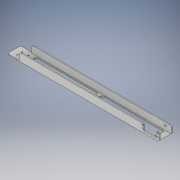
# Autodesk Inventor part: ArmProto1.2
Saved by Autodesk Inventor 2017 (Build 210142000, 142)
## iProperties
Created: 2017-09-30
Part Number: ArmProto1.2
Material: Generic
Document SubType Name: Modeling
Designer: User
Density: 1 g/cm^3
Appearance: Default
Author: User
Autodesk Inventor part; units mm, degrees
ref_plane "YZ Plane" through (0, 0, 0) normal (1, 0, 0) x (0, 1, 0)
ref_plane "XZ Plane" through (0, 0, 0) normal (0, 1, 0) x (-1, 0, 0)
ref_plane "XY Plane" through (0, 0, 0) normal (0, 0, 1) x (1, 0, 0)
sketch "Sketch1" plane through (0, 0, 0) normal (1, 0, 0) x (0, 1, 0)
  line L0 (0, 0) -> (25.4, 0)
  line L1 (25.4, 0) -> (25.4, -42.799)
  line L2 (25.4, -42.799) -> (0, -42.799)
  line L3 (0, -42.799) -> (0, 0)
  line L4 (25.4, -3.175) -> (3.175, -3.175)
  line L5 (3.175, -3.175) -> (3.175, -39.624)
  line L6 (3.175, -39.624) -> (25.4, -39.624)
  line L7 (25.4, -39.624) -> (25.4, -3.175)
  dimension "d0" = 25.4
  dimension "d1" = 42.799
  dimension "d2" = 22.225
  dimension "d3" = 36.449
  dimension "d4" = 3.175
  constraints: 16 end point, 4 parallel, 2 horizontal, 2 perpendicular, 1 point on line
  measures "d0" distance of L1.end L2.end
  measures "d1" distance of L0.end L1.end
  measures "d2" distance of L5.end L6.end
  measures "d3" distance of L4.end L5.end
  measures "d4" distance between parallel lines of L0 L4
extrude "Extrusion1" add sketch "Sketch1" along normal blind 495.3 contours L0 L1 L4 L5 L6 L2 L3
sketch "Sketch2" plane through (0, 0, 0) normal (0, 0, 1) x (1, 0, 0)
  line L0 (0, 25.4) -> (0, 0) projected
  line L1 (0, 0) -> (495.3, 0) projected
  line L2 (495.3, 25.4) -> (495.3, 0) projected
  line L3 (0, 25.4) -> (495.3, 25.4) projected
  line L4 (486.41, 25.4) -> (444.5, 25.4)
  line L5 (444.5, 25.4) -> (444.5, 6.35)
  line L6 (444.5, 6.35) -> (486.41, 6.35)
  line L7 (486.41, 6.35) -> (486.41, 25.4)
  circle A0 centre (490.2962, 21.2344) radius 2.413
  circle A1 centre (490.2962, 11.2344) radius 2.413
  circle A2 centre (440.7962, 21.2344) radius 2.413
  circle A3 centre (440.7962, 11.2344) radius 2.413
  dimension "d7" = 8.89
  dimension "d8" = 25.4
  dimension "d9" = 19.05
  dimension "d10" = 50.8
  dimension "d11" = 4.826
  dimension "d12" = 4.826
  dimension "d13" = 4.1656
  dimension "d14" = 10
  dimension "d15" = 4.826
  dimension "d16" = 4.826
  dimension "d26" = 5.0038
  dimension "d27" = 5.0038
  dimension "d28" = 49.5
  dimension "d29" = 49.5
  dimension "d30" = 10
  constraints: 8 end point, 4 centre point, 2 parallel, 1 horizontal, 1 perpendicular, 1 point on line
  measures "d7" distance between parallel lines of L2 L7
  measures "d8" distance of L2.start L1.end
  measures "d9" distance of L6.end L4.start
  measures "d10" distance between parallel lines of L2 L5
  measures "d11" diameter of A0
  measures "d12" diameter of A1
  measures "d13" distance from line of A0.centre L3
  measures "d14" distance of A1.centre A0.centre
  measures "d15" diameter of A2
  measures "d16" diameter of A3
  measures "d26" distance from line of L2 A0.centre
  measures "d27" distance from line of L2 A1.centre
  measures "d28" distance of A0.centre A2.centre
  measures "d29" distance of A1.centre A3.centre
  measures "d30" distance of A3.centre A2.centre
extrude "Extrusion2" cut sketch "Sketch2" against normal blind 12.7 contours L3 L7 L6 L5 | A0 | A1 | A2 | A3
sketch "Sketch3" plane through (0, 0, -42.799) normal (0, 0, -1) x (-1, 0, 0)
  line L0 (0, 0) -> (0, 25.4) projected
  line L1 (0, 25.4) -> (-495.3, 25.4) projected
  line L2 (-495.3, 0) -> (-495.3, 25.4) projected
  line L3 (0, 0) -> (-495.3, 0) projected
  circle A0 centre (-475.5896, 16.2306) radius 3.175
  point P0 (0, 0)
  dimension "d21" = 6.35
  dimension "d22" = 19.7104
  dimension "d23" = 9.1694
  constraints: 1 centre point
  measures "d21" diameter of A0
  measures "d22" distance from line of L2 A0.centre
  measures "d23" distance from line of L1 A0.centre
extrude "Extrusion3" cut sketch "Sketch3" against normal blind 12.7 contours A0
sketch "Sketch4" plane through (0, 0, -42.799) normal (0, -1, 0) x (1, 0, 0)
  line L0 (0, 42.799) -> (0, 0) projected
  line L1 (0, 42.799) -> (495.3, 42.799) projected
  line L2 (19.7866, 42.799) -> (19.7866, 30.6832)
  line L3 (19.7866, 42.799) -> (31.9024, 42.799) construction
  line L4 (0, 0) -> (495.3, 0) projected
  line L5 (19.7866, 0) -> (19.7866, 14.6812)
  line L6 (19.7866, 0) -> (34.4678, 0) construction
  circle A0 centre (19.7866, 30.6832) radius 1.8542
  circle A1 centre (19.7866, 14.6812) radius 1.8542
  line L7 (0, 14.6812) -> (40.2336, 14.6812)
  line L8 (0, 14.6812) -> (40.2336, 14.6812) construction
  circle A2 centre (40.2336, 14.6812) radius 1.8542
  circle A3 centre (40.2336, 30.6832) radius 1.8542
  dimension "d32" = 12.1158
  dimension "d33" = 90
  dimension "d34" = 14.6812
  dimension "d35" = 90
  dimension "d36" = 3.7084
  dimension "d37" = 3.7084
  dimension "d38" = 40.2336
  dimension "d40" = 3.7084
  constraints: 12 end point, 4 centre point, 3 coincident, 3 equal length, 3 horizontal, 3 perpendicular, 3 point on line
  measures "d32" distance of L2.start L2.end
  measures "d33" angle of L2 L3
  measures "d34" distance of L5.start L5.end
  measures "d35" angle of L6 L5
  measures "d36" diameter of A0
  measures "d37" diameter of A1
  measures "d38" distance of L7.start L7.end
  measures "d40" diameter of A2
extrude "Extrusion4" cut sketch "Sketch4" against normal blind 25.4 contours L7 L5 A1 | A1 L7 | A1 L5 L7 | A0 | A2 | A3
fillet "Fillet1" radius 3.175 3 edges at (495.3, 25.4, -1.5875) (486.41, 25.4, -1.5875) (444.5, 25.4, -1.5875)
fillet "Fillet2" radius 6.35 2 edges at (495.3, 25.4, -41.2115) (495.3, 0, -21.3995)
sketch "Sketch6" plane through (0, 0, 0) normal (0, 0, 1) x (1, 0, 0)
  circle A0 centre (440.7962, 11.2344) radius 2.413 projected
  circle A1 centre (490.2962, 11.2344) radius 2.413 projected
  circle A2 centre (490.2962, 21.2344) radius 2.413 projected
  circle A3 centre (440.7962, 21.2344) radius 2.413 projected
  arc A4 (488.95, 0) -> (495.3, 6.35) centre (488.95, 6.35) ccw projected
  line L0 (495.3, 22.225) -> (495.3, 6.35) projected
  arc A5 (495.3, 22.225) -> (492.125, 25.4) centre (492.125, 22.225) ccw projected
  line L1 (489.585, 25.4) -> (492.125, 25.4) projected
  arc A6 (489.585, 25.4) -> (486.41, 22.225) centre (489.585, 22.225) ccw projected
  line L2 (486.41, 22.225) -> (486.41, 6.35) projected
  line L3 (486.41, 6.35) -> (444.5, 6.35) projected
  line L4 (444.5, 6.35) -> (444.5, 22.225) projected
  arc A7 (444.5, 22.225) -> (441.325, 25.4) centre (441.325, 22.225) ccw projected
  line L5 (0, 25.4) -> (441.325, 25.4) projected
  line L6 (0, 25.4) -> (0, 0) projected
  line L7 (0, 0) -> (488.95, 0) projected
  line L8 (0, 25.4) -> (38.1, 25.4)
  line L9 (38.1, 25.4) -> (38.1, 3.175)
  line L10 (38.1, 3.175) -> (0, 3.175)
  line L11 (0, 3.175) -> (0, 25.4)
  dimension "d46" = 38.1
  dimension "d47" = 22.225
  constraints: 8 end point, 2 parallel, 1 horizontal, 1 perpendicular
  measures "d46" distance of L9.end L10.end
  measures "d47" distance of L8.end L9.end
extrude "Extrusion5" cut sketch "Sketch6" against normal blind 127 contours L6 L5 L9 L10
fillet "Fillet3" radius 6.35 4 edges at (38.1, 25.4, -1.5875) (38.1, 25.4, -41.2115) (0, 1.5875, 0) (0, 1.5875, -42.799)
sketch "Sketch7" plane through (488.95, 0, -42.799) normal (0, -1, 0) x (1, 0, 0)
  arc A0 (-488.95, 6.35) -> (-482.6, 0) centre (-482.6, 6.35) ccw projected
  line L0 (-482.6, 0) -> (0, 0) projected
  line L1 (0, 42.799) -> (0, 0) projected
  line L2 (-482.6, 42.799) -> (0, 42.799) projected
  arc A1 (-482.6, 42.799) -> (-488.95, 36.449) centre (-482.6, 36.449) ccw projected
  line L3 (-488.95, 36.449) -> (-488.95, 6.35) projected
  circle A2 centre (-448.7164, 30.6832) radius 1.8542 projected
  circle A3 centre (-469.1634, 14.6812) radius 1.8542 projected
  circle A4 centre (-469.1634, 30.6832) radius 1.8542 projected
  circle A5 centre (-448.7164, 14.6812) radius 1.8542 projected
  line L4 (-431.8, 36.449) -> (-228.6, 36.449)
  line L5 (-228.6, 36.449) -> (-228.6, 6.35)
  line L6 (-228.6, 6.35) -> (-431.8, 6.35)
  line L7 (-431.8, 6.35) -> (-431.8, 36.449)
  line L8 (-215.9, 36.449) -> (-12.7, 36.449)
  line L9 (-12.7, 36.449) -> (-12.7, 6.35)
  line L10 (-12.7, 6.35) -> (-215.9, 6.35)
  line L11 (-215.9, 6.35) -> (-215.9, 36.449)
  point P0 (-488.95, 42.799)
  dimension "d52" = 42.799
  dimension "d53" = 6.35
  dimension "d54" = 6.35
  dimension "d55" = 57.15
  dimension "d56" = 431.8
  dimension "d57" = 203.2
  dimension "d58" = 203.2
  dimension "d59" = 6.35
  dimension "d60" = 6.35
  dimension "d61" = 12.7
  constraints: 16 end point, 4 parallel, 2 horizontal, 2 perpendicular
  measures "d52" distance of L1.start L0.end
  measures "d53" distance between parallel lines of L2 L4
  measures "d54" distance between parallel lines of L0 L6
  measures "d55" distance between parallel lines of L3 L7
  measures "d56" distance between parallel lines of L1 L7
  measures "d57" distance of L4.start L4.end
  measures "d58" distance of L8.start L8.end
  measures "d59" distance between parallel lines of L2 L8
  measures "d60" distance between parallel lines of L0 L10
  measures "d61" distance between parallel lines of L5 L11
extrude "Extrusion6" cut sketch "Sketch7" against normal blind 127 contours L4 L5 L6 L7 | L8 L9 L10 L11
fillet "Fillet4" radius 6.35 8 edges at (260.35, 1.5875, -6.35) (57.15, 1.5875, -6.35) (57.15, 1.5875, -36.449) (273.05, 1.5875, -36.449) (273.05, 1.5875, -6.35) (260.35, 1.5875, -36.449) (476.25, 1.5875, -36.449) (476.25, 1.5875, -6.35)
equation "\"d12\" = d11"
equation "\"d15\" = d11"
equation "\"d16\" = d11"
equation "\"d27\" = d26"
equation "\"d29\" = d28"
equation "\"d30\" = d14"
equation "\"d58\" = d57"
body "Solid1"
